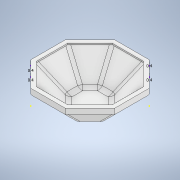
# Autodesk Inventor part: trail 6.1
Saved by Autodesk Inventor 2020.2 (Build 242310000, 310)
## iProperties
Created: 2020-02-13
Part Number: trail 6.1
Material: PVC, Unplasticized
Document SubType Name: Modeling
Designer: lenovo
Density: 1.29 g/cm^3
Appearance: Smooth - White
Author: lenovo
Autodesk Inventor part; units mm, degrees
ref_plane "YZ Plane" through (0, 0, 0) normal (1, 0, 0) x (0, 1, 0)
ref_plane "XZ Plane" through (0, 0, 0) normal (0, 1, 0) x (-1, 0, 0)
ref_plane "XY Plane" through (0, 0, 0) normal (0, 0, 1) x (1, 0, 0)
sketch "Sketch1" plane through (0, 0, 0) normal (0, 1, 0) x (-1, 0, 0)
  line L0 (-62.7534, -151.5) -> (-151.5, -62.7534)
  line L1 (-151.5, -62.7534) -> (-151.5, 62.7534)
  line L2 (-151.5, 62.7534) -> (-62.7534, 151.5)
  line L3 (-62.7534, 151.5) -> (62.7534, 151.5)
  line L4 (62.7534, 151.5) -> (151.5, 62.7534)
  line L5 (151.5, 62.7534) -> (151.5, -62.7534)
  line L6 (151.5, -62.7534) -> (62.7534, -151.5)
  line L7 (62.7534, -151.5) -> (-62.7534, -151.5)
  point P0 (0, 0)
  point P1 (0, 0)
  dimension "d0" = 303
  constraints: 16 end point, 1 coincident, 17 other
  measures "d0" distance between parallel lines of L3 L7
extrude "Extrusion1" add sketch "Sketch1" along normal blind 100
sketch "Sketch2" plane through (0, 100, 0) normal (0, 1, 0) x (1, 0, 0)
  line L0 (-136.5, 56.5402) -> (-56.5402, 136.5)
  line L1 (-56.5402, 136.5) -> (56.5402, 136.5)
  line L2 (56.5402, 136.5) -> (136.5, 56.5402)
  line L3 (136.5, 56.5402) -> (136.5, -56.5402)
  line L4 (136.5, -56.5402) -> (56.5402, -136.5)
  line L5 (56.5402, -136.5) -> (-56.5402, -136.5)
  line L6 (-56.5402, -136.5) -> (-136.5, -56.5402)
  line L7 (-136.5, -56.5402) -> (-136.5, 56.5402)
  point P0 (0, 0)
  point P1 (0, 0)
  dimension "d3" = 273
  constraints: 16 end point, 1 coincident, 17 other
  measures "d3" distance between parallel lines of L3 L7
extrude "Extrusion2" cut sketch "Sketch2" against normal blind 85
chamfer "Chamfer1" distance 80 angle 45 8 edges at (0, 15, 136.5) (96.5201, 15, 96.5201) (-96.5201, 15, 96.5201) (136.5, 15, 0) (96.5201, 15, -96.5201) (0, 15, -136.5) (-96.5201, 15, -96.5201) (-136.5, 15, 0)
chamfer "Chamfer2" distance 80 angle 45 8 edges at (-107.1267, 0, -107.1267) (0, 0, -151.5) (-151.5, 0, 0) (107.1267, 0, -107.1267) (151.5, 0, 0) (107.1267, 0, 107.1267) (0, 0, 151.5) (-107.1267, 0, 107.1267)
fillet "Fillet1" radius 25 16 edges at (46.1848, 40, 111.5) (111.5, 40, 46.1848) (111.5, 40, -46.1848) (-46.1848, 40, 111.5) (-111.5, 40, 46.1848) (46.1848, 40, -111.5) (-46.1848, 40, -111.5) (-111.5, 40, -46.1848) (-50.5581, 0, -50.5581) (0, 0, -71.5) (-71.5, 0, 0) (-50.5581, 0, 50.5581) (0, 0, 71.5) (50.5581, 0, 50.5581) (71.5, 0, 0) (50.5581, 0, -50.5581)
fillet "Fillet2" radius 25 16 edges at (39.9716, 55, 96.5) (96.5, 55, 39.9716) (96.5, 55, -39.9716) (-39.9716, 55, 96.5) (39.9716, 55, -96.5) (-39.9716, 55, -96.5) (-96.5, 55, -39.9716) (-96.5, 55, 39.9716) (-56.5, 15, 0) (-39.9515, 15, 39.9515) (-39.9515, 15, -39.9515) (0, 15, -56.5) (0, 15, 56.5) (39.9515, 15, 39.9515) (56.5, 15, 0) (39.9515, 15, -39.9515)
sketch "Sketch3" plane through (62.7534, 81.319, -151.5) normal (0.7071, 0, -0.7071) x (-0.7071, 0, -0.7071)
  circle A0 centre (-10, 7.5) radius 2
  point P0 (-62.7534, -81.319)
  dimension "d14" = 4
  constraints: 1 centre point
  measures "d14" diameter of A0
sketch "Sketch4" plane through (-62.7534, 81.319, 151.5) normal (-0.7071, 0, 0.7071) x (0.7071, 0, 0.7071)
  circle A0 centre (-115, 7.5) radius 2
  point P0 (-62.7534, -81.319)
  dimension "d15" = 4
  constraints: 1 centre point
  measures "d15" diameter of A0
sketch "Sketch5" plane through (62.7534, 81.319, -151.5) normal (0.7071, 0, -0.7071) x (-0.7071, 0, -0.7071)
  circle A0 centre (-62.755, 9.34) radius 2
  point P0 (-62.7534, -81.319)
  dimension "d16" = 4
  constraints: 1 centre point
  measures "d16" diameter of A0
sketch "Sketch6" plane through (-62.7534, 81.319, 151.5) normal (-0.7071, 0, 0.7071) x (0.7071, 0, 0.7071)
  circle A0 centre (-62.755, 9.34) radius 2
  point P0 (-62.7534, -81.319)
  dimension "d17" = 4
  constraints: 1 centre point
  measures "d17" diameter of A0
body "Solid1"
